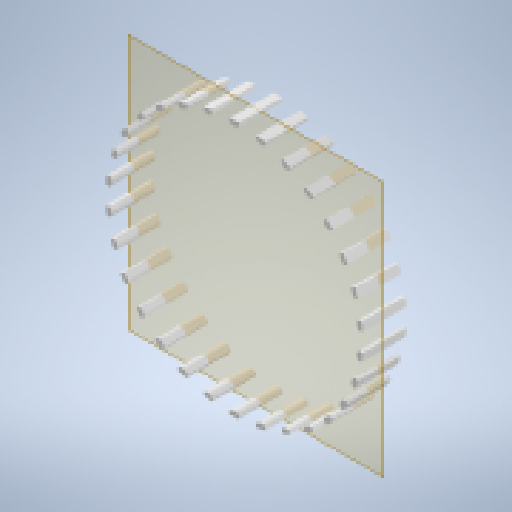
# Autodesk Inventor part: 1
Saved by Autodesk Inventor 2024 (Build 280153000, 153)
## iProperties
Created: 2023-11-21
Part Number: 1
Material: Ogólny
Document SubType Name: Modeling
Designer: Wojciech
Density: 1 g/cm^3
Appearance: Domyślna
Author: Wojciech
Autodesk Inventor part; units mm, degrees
ref_plane "YZ Plane" through (0, 0, 0) normal (1, 0, 0) x (0, 1, 0)
ref_plane "XZ Plane" through (0, 0, 0) normal (0, 1, 0) x (-1, 0, 0)
ref_plane "XY Plane" through (0, 0, 0) normal (0, 0, 1) x (1, 0, 0)
ref_plane "Płaszczyzna konstrukcyjna1" through (0, 0, -41) normal (0, 0, 1) x (1, 0, 0)
sketch "Szkic1" plane through (0, 0, -41) normal (0, 0, 1) x (1, 0, 0)
  line L0 (33.0313, -4.4652) -> (29.7621, -3.7703) projected
  spline S0 degree 3 poles (34.4436, -5.6103) (34.3457, -5.3896) (34.1853, -5.1565) (33.8544, -4.838) (33.6651, -4.7033) (33.3685, -4.5662) (33.2791, -4.5324) (33.1885, -4.5053) knots 1.429886 1.429886 1.429886 1.429886 1.512632 1.512632 1.579596 1.579596 1.606867 1.606867 1.606867 1.606867 projected
  spline S1 degree 3 poles (34.6264, -7.3601) (34.6901, -7.0607) (34.7087, -6.7247) (34.628, -6.1237) (34.554, -5.859) (34.4436, -5.6103) knots 0 0 0 0 0.119776 0.119776 0.213474 0.213474 0.213474 0.213474 projected
  spline S2 degree 3 poles (33.7477, -8.8843) (33.9497, -8.7019) (34.1249, -8.4902) (34.4431, -7.974) (34.5628, -7.6595) (34.6264, -7.3601) knots 1.200903 1.200903 1.200903 1.200903 1.294601 1.294601 1.414377 1.414377 1.414377 1.414377 projected
  spline S3 degree 3 poles (32.1517, -9.3832) (32.2455, -9.3953) (32.3409, -9.4007) (32.6676, -9.3962) (32.8953, -9.3501) (33.3272, -9.1937) (33.5685, -9.046) (33.7477, -8.8843) knots 0.979714 0.979714 0.979714 0.979714 1.006985 1.006985 1.073949 1.073949 1.156696 1.156696 1.156696 1.156696 projected
  line L1 (28.7226, -8.661) -> (31.9918, -9.3559) projected
  arc A0 (33.1885, -4.5053) -> (33.0313, -4.4652) centre (32.6155, -6.4215) ccw projected
  arc A1 (31.9918, -9.3559) -> (32.1517, -9.3832) centre (32.4076, -7.3996) ccw projected
  line L2 (33.1885, -4.5053) -> (32.1517, -9.3832) projected
  line L3 (33.9207, -2.5) -> (33.9207, 2.5) construction
  line L4 (33.4, 2.4934) -> (33.4, -2.4934) projected
  circle A2 centre (0, 0) radius 35.3971
  line L5 (29.8957, -2.5) -> (33.2379, -2.5) projected
  line L6 (29.8957, -2.5) -> (29.7621, -3.7703)
  line L7 (35.3971, 0) -> (34.6264, -7.3601)
  line L8 (29.8289, -3.1351) -> (35.0117, -3.68)
  line L9 (35.0117, -3.68) -> (35.2032, -3.7001)
  line L10 (35.0117, -3.68) -> (35.1367, -2.4866)
  line L11 (35.1367, -2.4866) -> (35.3084, -2.5045)
  line L12 (34.8858, -4.8734) -> (35.0574, -4.8915)
  line L13 (35.1367, -2.4866) -> (34.3857, -2.4079)
  line L14 (34.3857, -2.4079) -> (34.2602, -3.601)
  arc A3 (34.3857, -2.4079) -> (33.798, -3.5524) centre (35.5689, -3.7386) ccw
  line L15 (34.8858, -4.8734) -> (34.1348, -4.7941)
  arc A4 (33.798, -3.5524) -> (34.1348, -4.7941) centre (35.5689, -3.7386) ccw
  line L16 (34.1348, -4.7941) -> (35.0584, -4.8916)
  circle A5 centre (0, 0) radius 52.5
  circle A6 centre (0, 0) radius 72.5
  point P0 (35.0575, -4.8915)
  dimension "d0" = 70.7942
  dimension "d1" = 1.2
  dimension "d5" = 5.1829
  dimension "d7" = 105
  dimension "d8" = 145
  constraints: 22 end point, 7 point on circle, 5 centre point, 4 perpendicular, 4 symmetric about line, 3 coincident, 3 point on line, 2 midpoint, 1 concentric, 1 other
  measures "d0" diameter of A2
  measures "d1" distance of L8.end L10.end
  measures "d5" horizontal distance of L8.start L8.end
  measures "d7" diameter of A5
  measures "d8" diameter of A6
extrude "Wyciągnięcie proste1" add sketch "Szkic1" along normal mid plane 14 contours A3 L14 L8 | L8 L7 L15 A4 | L14 L13 L7 L8 | L7 L9 A2 L12 | L7 L11 A2 L9
pattern_circular "Szyk kołowy1" count 30 over 360 about axis through (0, 0, -10) along (0, 0, 1) of "Wyciągnięcie proste1"
